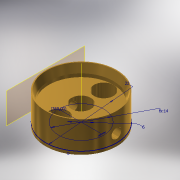
# Autodesk Inventor part: nozzle-base
Saved by Autodesk Inventor 2016 (Build 200138000, 138)
## iProperties
Created: 2015-05-09
Part Number: nozzle-base
Material: Brass, Soft Yellow
Document SubType Name: Modeling
Designer: ax
Mass: 15.995 g
Surface Area: 19.7226 cm^2
Volume: 1.88843 cm^3
Density: 8.47 g/cm^3
Appearance: Brass - Satin
dO: 22,000 mm
di: 6,000 mm
d2: 14,000 mm
d3: 4,000 ul
d5: 360,00 deg
d7: 8,500 mm
d8: 0,00 deg
dnozzle: 20,000 mm
d10: 3,500 mm
d11: 0,00 deg
d12: 0,700 mm
d13: 2,500 mm
d22: 0,000 mm
d23: 6,000 mm
d32: -11,000 mm
d33: 2,500 mm
d35: 11,000 mm
d36: 3,000 mm
d41: 24,000 mm
d42: 118,00 deg
deep: 5,000 mm
Author: ax
Autodesk Inventor part; units mm, degrees
ref_plane "XZ Plane" through (0, 0, 0) normal (0, 1, 0) x (-1, 0, 0)
ref_plane "XY Plane" through (0, 0, 0) normal (0, 0, 1) x (1, 0, 0)
sketch "Sketch1" plane through (0, 0, 0) normal (0, 0, 1) x (1, 0, 0)
  circle A0 centre (0, 0) radius 11
  circle A1 centre (0, 0) radius 3
  circle A2 centre (0, 0) radius 7 construction
  circle A3 centre (0, 0) radius 7 construction
  circle A4 centre (0, 0) radius 7 construction
  circle A5 centre (0, 0) radius 7 construction
  point P0 (-7, 0)
  point P1 (0, -7)
  point P2 (7, 0)
  point P3 (0, 7)
  dimension "d2" = 14
  dimension "dO" = 22
  dimension "di" = 6
  dimension "d5" = 360
  dimension "d22" = 0
  constraints: 5 coincident, 2 centre point, 2 horizontal alignment, 2 vertical alignment, 19 other
  measures "dO" diameter of A0
  measures "di" diameter of A1
  measures "d22" vertical distance of point (0, 0) point (-7, 0)
extrude "Extrusion1" add sketch "Sketch1" along normal blind 8.5
sketch "Sketch2" plane through (0, 0, 8.5) normal (0, 0, 1) x (1, 0, 0)
  circle A0 centre (0, 0) radius 10
  dimension "dnozzle" = 20
  constraints: 1 centre point, 1 coincident
  measures "dnozzle" diameter of A0
extrude "Extrusion2" cut sketch "Sketch2" against normal blind 3.5
chamfer "Chamfer1" distance 0.7 distance2 2.5 1 edges at (-10, 0, 8.5) measured on face at (-10.5, 0, 8.5)
hole "Hole2" at (0, -7, 0) at (0, 7, 0) direction (0, 0, 1) diameter 6 end through all
ref_plane "Work Plane2" through (-11, 0, 0) normal (1, 0, 0) x (0, 1, 0)
sketch "Sketch5" plane through (-11, 0, 0) normal (1, 0, 0) x (0, 1, 0)
  line L0 (-11, 0) -> (11, 0) projected
  point P0 (0, 0)
  point P1 (0, 2.5)
  dimension "d33" = 2.5
  dimension "d35" = 11
  measures "d33" distance from line of L0 point (0, 2.5)
  measures "d35" horizontal distance of L0.end point (0, 2.5)
hole "Hole3" at (-11, 0, 2.5) direction (1, 0, 0) diameter 3 depth 24 tip angle 118
extrude "Extrusion3" add sketch "Sketch1" against normal blind 1
equation "\"d2\" = 0.5 * dO + 0.5 * di"
equation "\"d33\" = -0.5 * d10 + 0.5 * d7"
equation "\"d35\" = 0.5 * dO"
equation "\"d32\" = -0.5 * dO"
equation "\"deep\" = d7 - d10"
equation "\"d7\" = 8.5"
equation "\"d10\" = 3.5"
body "Solid1"
